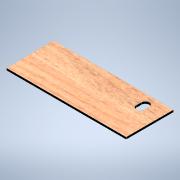
# Autodesk Inventor part: wood_front
Saved by Autodesk Inventor 2021 (Build 250183000, 183)
## iProperties
Created: 2021-08-17
Part Number: wood_front
Material: Generisch
Document SubType Name: Modeling
Designer: Tilman
Density: 1 g/cm^3
Appearance: Eloxiert - Schwarz
Author: Tilman
Autodesk Inventor part; units mm, degrees
ref_plane "YZ Plane" through (0, 0, 0) normal (1, 0, 0) x (0, 1, 0)
ref_plane "XZ Plane" through (0, 0, 0) normal (0, 1, 0) x (-1, 0, 0)
ref_plane "XY Plane" through (0, 0, 0) normal (0, 0, 1) x (1, 0, 0)
sketch "Skizze1" plane through (0, 0, 0) normal (0, 1, 0) x (-1, 0, 0)
  line L0 (0, 0) -> (-165.5, 0)
  line L1 (-165.5, 0) -> (-165.5, -65.5)
  line L2 (-165.5, -65.5) -> (0, -65.5)
  line L3 (0, -65.5) -> (0, 0)
  line L4 (-134.5, -45) -> (-134.5, -52)
  line L5 (-145.5, -52) -> (-145.5, -45)
  arc A0 (-145.5, -52) -> (-134.5, -52) centre (-140, -52) ccw
  arc A1 (-134.5, -45) -> (-145.5, -45) centre (-140, -45) ccw
  dimension "d0" = 165.5
  dimension "d1" = 65.5
  dimension "d8" = 11
  dimension "d9" = 7
  dimension "d10" = 13.5
  dimension "d11" = 20
  constraints: 12 end point, 4 point on circle, 3 parallel, 3 tangent, 2 centre point, 1 equal radius, 1 horizontal, 1 perpendicular, 1 vertical
  measures "d0" distance of L0.start L0.end
  measures "d1" distance of L2.end L0.start
  measures "d8" distance between parallel lines of L5 L4
  measures "d9" distance of L5.start L5.end
  measures "d10" distance from line of L2 A0.centre
  measures "d11" distance between parallel lines of L1 L5
extrude "Extrusion1" add sketch "Skizze1" along normal blind 3
